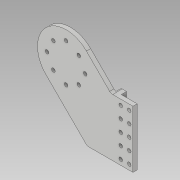
# Autodesk Inventor part: dynamixel_pro_frame_part3
Saved by Autodesk Inventor 2017 (Build 210142000, 142)
## iProperties
Part Number: dynamixel_pro_frame_part3
Material: Aluminium 6061
Document SubType Name: Modeling
Designer: Max
Density: 2.7 g/cm^3
Appearance: Vorgabe
Mass: 61.3934 g
Surface Area: 132.539 cm^2
Volume: 22.7383 cm^3
Author: Max
Autodesk Inventor part; units mm, degrees
ref_plane "YZ Plane" through (0, 0, 0) normal (1, 0, 0) x (0, 1, 0)
ref_plane "XZ Plane" through (0, 0, 0) normal (0, 1, 0) x (-1, 0, 0)
ref_plane "XY Plane" through (0, 0, 0) normal (0, 0, 1) x (1, 0, 0)
sketch "Skizze1" plane through (0, 0, 0) normal (0, 1, 0) x (-1, 0, 0)
  line L0 (0, 27) -> (0, -27)
  line L1 (0, 27) -> (20.8162, 27)
  line L2 (20.8162, 27) -> (43.9081, 50.0919)
  line L3 (0, -27) -> (43.1838, -27)
  line L4 (43.1838, -27) -> (82.0919, 11.9081)
  arc A0 (82.0919, 11.9081) -> (43.9081, 50.0919) centre (63, 31) ccw
  point P0 (0, 0)
  point P1 (0, 0)
  dimension "d43" = 54
  dimension "d44" = 135
  dimension "d46" = 31
  dimension "d47" = 63
  dimension "d48" = 54
  constraints: 10 end point, 2 horizontal, 2 point on circle, 2 tangent, 1 centre point, 1 coincident, 1 midpoint, 1 parallel, 1 vertical
  measures "d43" distance of L0.start L0.end
  measures "d44" angle of L2 L1
  measures "d46" vertical distance of point (0, 0) A0.centre
  measures "d47" distance from line of L0 A0.centre
  measures "d48" distance between parallel lines of L4 L2
extrude "Extrusion1" add sketch "Skizze1" along normal blind 4
sketch "Skizze5" plane through (0, 4, 0) normal (0, 1, 0) x (1, 0, 0)
  line L0 (0, -27) -> (0, 27) projected
  line L1 (0, 27) -> (-43.1838, 27) projected
  line L2 (-43.1838, 27) -> (-82.0919, -11.9081) projected
  arc A0 (-82.0919, -11.9081) -> (-43.9081, -50.0919) centre (-63, -31) ccw projected
  line L3 (-43.9081, -50.0919) -> (-20.8162, -27) projected
  line L4 (-20.8162, -27) -> (0, -27) projected
  line L5 (-20, -27) -> (-15, -27)
  line L6 (-15, -27) -> (-15, 27)
  line L7 (-15, 27) -> (-20, 27)
  line L8 (-20, 27) -> (-20, -27)
  dimension "d49" = 5
  dimension "d50" = 15
  constraints: 8 end point, 2 parallel, 2 point on line, 1 horizontal, 1 perpendicular
  measures "d49" distance between parallel lines of L8 L6
  measures "d50" distance between parallel lines of L0 L6
extrude "Extrusion4" add sketch "Skizze5" along normal blind 5 contours L4 L8 L1 L6
sketch "Skizze6" plane through (0, 4, 0) normal (0, 1, 0) x (1, 0, 0)
  point P0 (0, 0)
  point P1 (-3.5, 0)
  dimension "d51" = 3.5
  measures "d51" distance of point (-3.5, 0) point (0, 0)
hole "Bohrung1" at (-3.5, 4, 0) direction (0, -1, 0) diameter 3.4 end through all clearance for "Inbusschraube ISO 4762" size "M3" standard "ISO"
pattern_linear "Rechteckige Anordnung1" count 5 spacing 11 along (0, 0, -1) count 2 spacing 8 along (-1, 0, 0) of "Bohrung1" first direction both ways yes
sketch "Skizze7" plane through (0, 0, 0) normal (0, -1, 0) x (1, 0, 0)
  line L0 (-51, 43) -> (-75, 43)
  line L1 (-75, 43) -> (-75, 19)
  line L2 (-75, 19) -> (-51, 19)
  line L3 (-51, 19) -> (-51, 43)
  line L4 (-51, 43) -> (-75, 19) construction
  line L5 (-63, 63.2011) -> (-63, 8.0055) construction
  circle A0 centre (-63, 31) radius 18
  line L6 (-63, 26.0548) -> (-63, -18.8231) construction
  line L7 (-38.3888, 31) -> (-81.0377, 31) construction
  arc A1 (-43.9081, 50.0919) -> (-82.0919, 11.9081) centre (-63, 31) ccw projected
  line L8 (-51, 19) -> (-75, 43) construction
  point P0 (-63, 13)
  point P1 (-81, 31)
  point P2 (-63, 13)
  point P3 (-63, 31)
  point P4 (-45, 31)
  point P5 (-63, 49)
  dimension "d32" = 24
  dimension "d33" = 24
  dimension "d35" = 36
  constraints: 18 end point, 9 point on line, 5 point on circle, 2 coincident, 2 horizontal, 2 midpoint, 2 parallel, 1 centre point, 1 perpendicular, 1 vertical
  measures "d32" distance of L1.end L2.end
  measures "d33" distance of L0.end L1.end
  measures "d35" diameter of A0
hole "Bohrung2" at (-63, 0, 13) at (-81, 0, 31) at (-51, 0, 19) at (-75, 0, 19) at (-75, 0, 43) at (-51, 0, 43) at (-63, 0, 49) at (-45, 0, 31) direction (0, 1, 0) diameter 3.4 end through all clearance for "Inbusschraube ISO 4762" size "M3" standard "ISO"
fillet "Rundung1" radius 4 2 edges at (-43.1838, 2, -27) (-20.8162, 2, 27)
equation "\"d48\" = d43"
